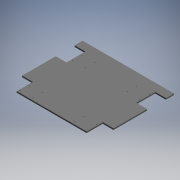
# Autodesk Inventor part: Gen 2.0 rev mecanums base plate
Saved by Autodesk Inventor 2019 (Build 230136000, 136)
## iProperties
Part Number: Gen 2.0 rev mecanums base plate
Material: Generic
Document SubType Name: Modeling
Designer: Delta
Appearance: Default
Author: Delta
Autodesk Inventor part; units mm, degrees
ref_plane "YZ Plane" through (0, 0, 0) normal (1, 0, 0) x (0, 1, 0)
ref_plane "XZ Plane" through (0, 0, 0) normal (0, 1, 0) x (-1, 0, 0)
ref_plane "XY Plane" through (0, 0, 0) normal (0, 0, 1) x (1, 0, 0)
sketch "Sketch1" plane through (0, 0, 0) normal (0, 1, 0) x (-1, 0, 0)
  line L0 (0, 0) -> (431.8, 0)
  line L1 (431.8, 0) -> (431.8, 361.95)
  line L2 (431.8, 361.95) -> (0, 361.95)
  line L3 (0, 361.95) -> (0, 0)
  dimension "d0" = 431.8
  dimension "d1" = 361.95
  constraints: 8 end point, 2 parallel, 1 horizontal, 1 perpendicular
  measures "d0" distance of L1.end L2.end
  measures "d1" distance of L0.end L1.end
extrude "Extrusion1" add sketch "Sketch1" along normal blind 6.35
sketch "Sketch3" plane through (0, 6.35, 0) normal (0, 1, 0) x (1, 0, 0)
  line L0 (-431.8, 0) -> (-431.8, -361.95) projected
  line L1 (-431.8, -361.95) -> (-381, -361.95)
  line L2 (-381, -361.95) -> (-381, -285.75)
  line L3 (-381, -285.75) -> (-431.8, -285.75)
  line L4 (-431.8, -285.75) -> (-431.8, -361.95)
  line L5 (-431.8, -38.1) -> (-381, -38.1)
  line L6 (-381, -38.1) -> (-381, -127)
  line L7 (-381, -127) -> (-431.8, -127)
  line L8 (-431.8, -127) -> (-431.8, -38.1)
  line L9 (0, -361.95) -> (0, 0) projected
  line L10 (0, -38.1) -> (-50.8, -38.1)
  line L11 (-50.8, -38.1) -> (-50.8, -127)
  line L12 (-50.8, -127) -> (0, -127)
  line L13 (0, -127) -> (0, -38.1)
  line L14 (0, -361.95) -> (-50.8, -361.95)
  line L15 (-50.8, -361.95) -> (-50.8, -285.75)
  line L16 (-50.8, -285.75) -> (0, -285.75)
  line L17 (0, -285.75) -> (0, -361.95)
  line L18 (0, 0) -> (-431.8, 0) projected
  dimension "d11" = 76.2
  dimension "d12" = 88.9
  dimension "d13" = 127
  dimension "d14" = 50.8
  dimension "d15" = 50.8
  constraints: 32 end point, 8 parallel, 7 point on line, 4 horizontal, 4 perpendicular
  measures "d11" distance between parallel lines of L1 L3
  measures "d12" distance between parallel lines of L7 L5
  measures "d13" distance between parallel lines of L7 L18
  measures "d14" distance between parallel lines of L2 L4
  measures "d15" distance between parallel lines of L17 L15
extrude "Extrusion3" cut sketch "Sketch3" against normal blind 6.35
sketch "Sketch4" plane through (0, 6.35, 0) normal (0, 1, 0) x (1, 0, 0)
  line L0 (0, 0) -> (-431.8, 0) projected
  line L1 (-381, -38.1) -> (-381, -127) projected
  line L2 (-381, -285.75) -> (-381, -361.95) projected
  line L3 (-381, -361.95) -> (-50.8, -361.95) projected
  point P0 (-375.0056, -60.8076)
  point P1 (-375.0056, -103.8098)
  point P2 (-314.0964, -60.8076)
  point P3 (-314.0964, -103.8098)
  point P4 (-375.0056, -351.4598)
  point P5 (-375.0056, -308.4576)
  point P6 (-314.0964, -351.4598)
  point P7 (-314.0964, -308.4576)
  dimension "d18" = 60.8076
  dimension "d19" = 5.9944
  dimension "d20" = 103.8098
  dimension "d21" = 5.9944
  dimension "d22" = 66.9036
  dimension "d23" = 60.8076
  dimension "d24" = 103.8098
  dimension "d25" = 66.9036
  dimension "d26" = 5.9944
  dimension "d27" = 10.4902
  dimension "d28" = 5.9944
  dimension "d29" = 53.4924
  dimension "d30" = 66.9036
  dimension "d31" = 66.9036
  dimension "d32" = 10.4902
  dimension "d33" = 53.4924
  measures "d18" distance from line of L0 point (-375.006, -60.808)
  measures "d19" distance from line of point (-375.006, -60.808) L1
  measures "d20" distance from line of L0 point (-375.006, -103.81)
  measures "d21" distance from line of L1 point (-375.006, -103.81)
  measures "d22" distance from line of L1 point (-314.096, -60.808)
  measures "d23" distance from line of point (-314.096, -60.808) L0
  measures "d24" distance from line of L0 point (-314.096, -103.81)
  measures "d25" distance from line of L1 point (-314.096, -103.81)
  measures "d26" distance from line of L2 point (-375.006, -351.46)
  measures "d27" distance from line of L3 point (-375.006, -351.46)
  measures "d28" distance from line of L2 point (-375.006, -308.458)
  measures "d29" distance from line of L3 point (-375.006, -308.458)
  measures "d30" distance from line of L2 point (-314.096, -351.46)
  measures "d31" distance from line of L2 point (-314.096, -308.458)
  measures "d32" distance from line of L3 point (-314.096, -351.46)
  measures "d33" distance from line of L3 point (-314.096, -308.458)
hole "Hole1" at (-375.0056, 6.35, 60.8076) at (-375.0056, 6.35, 103.8098) at (-314.0964, 6.35, 60.8076) at (-314.0964, 6.35, 103.8098) at (-375.0056, 6.35, 351.4598) at (-375.0056, 6.35, 308.4576) at (-314.0964, 6.35, 351.4598) at (-314.0964, 6.35, 308.4576) direction (0, -1, 0) diameter 3.81 end through all
ref_plane "Work Plane1" through (-215.9, 0, 285.75) normal (1, 0, 0) x (0, 0, -1)
mirror "Mirror1" about plane through (-215.9, 0, 285.75) normal (1, 0, 0) of "Hole1"
equation "\"d18\" = d23"
equation "\"d19\" = d21"
equation "\"d22\" = d25"
equation "\"d24\" = d20"
equation "\"d26\" = d21"
equation "\"d27\" = d32"
equation "\"d28\" = d21"
equation "\"d30\" = d25"
equation "\"d31\" = d25"
equation "\"d33\" = d29"
body "Solid1"
